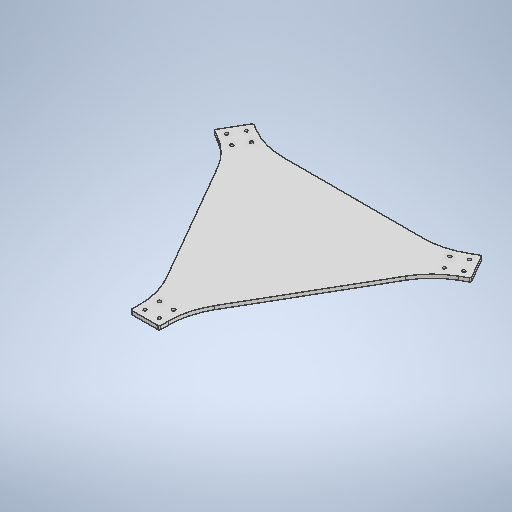
# Autodesk Inventor part: RT_FRM_MC_004_BasePlateTop
Saved by Autodesk Inventor 2025.3 (Build 293356000, 356)
## iProperties
Created: 2026-05-11
Part Number: RT_FRM_MC_004_BasePlateTop
Material: Generic
Document SubType Name: Modeling
Designer: louis
Density: 1 g/cm^3
Appearance: Default
Author: louis
Autodesk Inventor part; units mm, degrees
ref_plane "YZ Plane" through (0, 0, 0) normal (1, 0, 0) x (0, 1, 0)
ref_plane "XZ Plane" through (0, 0, 0) normal (0, 1, 0) x (-1, 0, 0)
ref_plane "XY Plane" through (0, 0, 0) normal (0, 0, 1) x (1, 0, 0)
sketch "Sketch1" plane through (0, 0, 0) normal (0, 1, 0) x (-1, 0, 0)
  line L0 (0, 379.282) -> (328.4679, -189.641) construction
  line L1 (328.4679, -189.641) -> (-328.4679, -189.641) construction
  line L2 (-328.4679, -189.641) -> (0, 379.282) construction
  line L3 (248.4679, -189.641) -> (288.4679, -120.359)
  line L4 (-248.4679, -189.641) -> (-288.4679, -120.359)
  line L5 (40, 310) -> (-40, 310)
  line L6 (164.2339, 94.8205) -> (0, 0) construction
  line L7 (0, -189.641) -> (0, 0) construction
  line L8 (0, 0) -> (-164.2339, 94.8205) construction
  line L9 (288.4679, -120.359) -> (40, 310)
  line L10 (-40, 310) -> (-288.4679, -120.359)
  line L11 (-248.4679, -189.641) -> (248.4679, -189.641)
  line L12 (288.4679, -120.359) -> (248.4679, -189.641)
  line L13 (248.4679, -189.641) -> (317.7499, -229.641)
  line L14 (317.7499, -229.641) -> (357.7499, -160.359)
  line L15 (357.7499, -160.359) -> (288.4679, -120.359)
  line L16 (-288.4679, -120.359) -> (-248.4679, -189.641)
  line L17 (-248.4679, -189.641) -> (-317.7499, -229.641)
  line L18 (-317.7499, -229.641) -> (-357.7499, -160.359)
  line L19 (-357.7499, -160.359) -> (-288.4679, -120.359)
  line L20 (-40, 310) -> (40, 310)
  line L21 (40, 310) -> (40, 390)
  line L22 (40, 390) -> (-40, 390)
  line L23 (-40, 390) -> (-40, 310)
  line L24 (-357.7499, 390) -> (-357.7499, -229.641) construction
  line L25 (-357.7499, -229.641) -> (357.7499, -229.641) construction
  line L26 (357.7499, -229.641) -> (357.7499, 390) construction
  line L27 (357.7499, 390) -> (-357.7499, 390) construction
  circle A0 centre (0, 0) radius 300 construction
  dimension "d4" = 80
  dimension "d6" = 80
  dimension "d7" = 80
  dimension "d8" = 80
  dimension "d10" = 390
  dimension "d13" = 619.641
  dimension "d14" = 715.4998
  dimension "d28" = 600
  constraints: 56 end point, 10 point on line, 9 parallel, 7 perpendicular, 4 equal length, 3 midpoint, 3 symmetric about line, 2 coincident, 2 collinear, 2 vertical, 1 centre point, 1 horizontal
  measures "d4" distance of L3.start L3.end
  measures "d6" distance of L13.end L3.start
  measures "d7" distance of L4.start L17.end
  measures "d8" distance of L21.end L5.start
  measures "d10" distance from line of point (0, 0) L18
  measures "d13" distance of L24.start L24.end
  measures "d14" distance of L26.end L24.start
  measures "d28" diameter of A0
extrude "Extrusion1" add sketch "Sketch1" along normal blind 10
fillet "Fillet1" radius 200 6 edges at (-40, 5, 310) (40, 5, 310) (-288.4679, 5, -120.359) (-248.4679, 5, -189.641) (248.4679, 5, -189.641) (288.4679, 5, -120.359)
fillet "Fillet2" radius 4 6 edges at (-40, 5, 390) (40, 5, 390) (-357.7499, 5, -160.359) (-317.7499, 5, -229.641) (317.7499, 5, -229.641) (357.7499, 5, -160.359)
sketch "Sketch2" plane through (0, 0, 0) normal (0, -1, 0) x (1, 0, 0)
  line L0 (40, 390) -> (-40, 390) construction
  line L1 (-40, 390) -> (-40, 310) construction
  line L2 (-40, 310) -> (40, 310) construction
  line L3 (40, 310) -> (40, 390) construction
  line L4 (-40, 363.5898) -> (-40, 386) construction
  line L5 (-36, 390) -> (36, 390) construction
  line L6 (40, 386) -> (40, 363.5898) construction
  line L7 (0, 390) -> (0, 310) construction
  line L8 (40, 350) -> (-40, 350) construction
  point P0 (0, 0)
  point P1 (20, 370)
  point P2 (-20, 370)
  point P3 (-20, 330)
  point P4 (20, 330)
  dimension "d15" = 80
  dimension "d16" = 40
  dimension "d17" = 40
  constraints: 12 end point, 4 midpoint, 3 collinear, 3 symmetric about line, 2 parallel, 1 horizontal, 1 perpendicular
  measures "d15" distance of L2.end L0.start
  measures "d16" distance of point (20, 330) point (20, 370)
  measures "d17" distance of point (20, 370) point (-20, 370)
hole "Hole1" at (20, 0, 370) at (-20, 0, 370) at (-20, 0, 330) at (20, 0, 330) direction (0, 1, 0) diameter 9 end through all countersink diameter 17.3 countersink angle 90 clearance for "Flat Head Machine Screw" size "M8" standard "Ansi Metric M Profile"
pattern_circular "Circular Pattern1" count 3 over 360 about axis through (0, -10, 0) along (0, 1, 0) of "Hole1"
body "Solid1"
